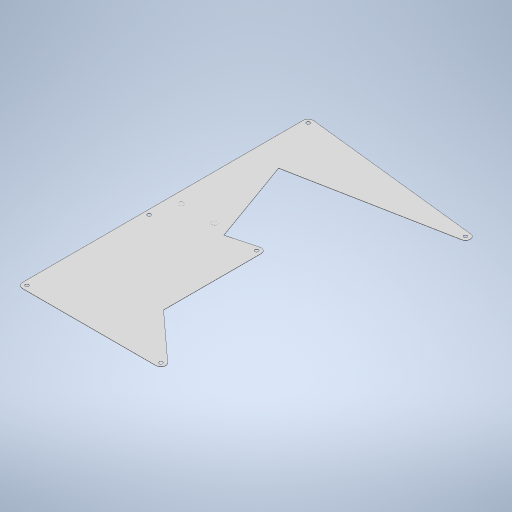
# Autodesk Inventor part: base_main_pcb_full
Saved by Autodesk Inventor 2024 (Build 280153000, 153)
## iProperties
Created: 2026-03-21
Part Number: base_main_pcb_full
Material: Generic
Document SubType Name: Modeling
Designer: schar
Density: 1 g/cm^3
Appearance: Default
Author: schar
Autodesk Inventor part; units mm, degrees
ref_plane "YZ Plane" through (0, 0, 0) normal (1, 0, 0) x (0, 1, 0)
ref_plane "Work Plane1" through (-205, 0.2, 0) normal (0, 1, 0) x (1, 0, 0)
sketch "Sketch1" plane through (-205, 0.2, 0) normal (0, 1, 0) x (1, 0, 0)
  circle A0 centre (172.5, -37.3) radius 1.675 projected
  circle A1 centre (172.5, -37.3) radius 4.5
  circle A2 centre (172.5, -37.3) radius 1.675
  circle A3 centre (7.5, -19) radius 1.675 projected
  circle A4 centre (7.5, -19) radius 4.5
  circle A5 centre (7.5, -19) radius 1.675
  circle A6 centre (86.5, -146.2) radius 1.675 projected
  circle A7 centre (86.5, -146.2) radius 4.5
  circle A8 centre (86.5, -146.2) radius 1.675
  circle A9 centre (7.5, -167.45) radius 1.675 projected
  circle A10 centre (7.5, -167.45) radius 4.5
  circle A11 centre (7.5, -167.45) radius 1.675
  circle A12 centre (7.5, -281.46) radius 1.675 projected
  circle A13 centre (7.5, -281.46) radius 4.5
  circle A14 centre (7.5, -281.46) radius 1.675
  circle A15 centre (132.5, -281.46) radius 1.675 projected
  circle A16 centre (132.5, -281.46) radius 4.5
  circle A17 centre (132.5, -281.46) radius 1.675
  line L0 (132.5, -285.96) -> (7.5, -285.96)
  line L1 (3, -281.46) -> (3, -167.45)
  line L2 (135.7704, -278.369) -> (10.5327, -164.1254)
  line L3 (91, -146.2) -> (91, -237.5288)
  line L4 (84.825, -142.0234) -> (6.3328, -163.104)
  line L5 (91, -237.5288) -> (10.5327, -164.1254)
  line L6 (12, -19) -> (58.7973, -149.0136)
  line L7 (3, -19) -> (3, -167.45)
  line L8 (172.5, -41.8) -> (30.084, -69.2416)
  line L9 (172.5, -32.8) -> (8.061, -14.5351)
  point P0 (205, 0)
  dimension "d1" = 9
  dimension "d2" = 9
  dimension "d3" = 9
  dimension "d4" = 9
  dimension "d5" = 9
  dimension "d6" = 9
  constraints: 20 end point, 14 point on circle, 12 centre point, 12 coincident, 6 tangent, 2 point on line, 1 concentric, 1 parallel, 1 perpendicular, 1 vertical
  measures "d1" diameter of A1
  measures "d2" diameter of A4
  measures "d3" diameter of A7
  measures "d4" diameter of A10
  measures "d5" diameter of A13
  measures "d6" diameter of A16
extrude "Extrusion1" add sketch "Sketch1" along normal blind 0.2 contours A1 | A1 L8 L6 A4 L9 | A4 | L6 L4 A10 L7 A4 | L4 A7 L3 L2 A10 | A10 | A10 L2 A16 L0 A13 L1 | A7 | A13 | A16 L2 picked at (134.365, -278.4554)
ref_plane "Work Plane2" through (-205, 0.4, 0) normal (0, 1, 0) x (1, 0, 0)
sketch "Sketch3" plane through (-205, 0.2, 0) normal (0, -1, 0) x (1, 0, 0)
  line L0 (3, 19) -> (3, 281.46) projected
  line L1 (3, 143.5142) -> (56.8178, 143.5142)
  line L2 (58.7973, 149.0136) -> (30.084, 69.2416) projected
  circle A0 centre (13.4848, 143.5142) radius 2.5
  circle A1 centre (44.4406, 143.5142) radius 2.5
  point P0 (205, 0)
  dimension "d11" = 5
  dimension "d12" = 5
  constraints: 4 point on line, 2 centre point, 2 end point, 1 horizontal
  measures "d11" diameter of A0
  measures "d12" diameter of A1
extrude "Extrusion2" add sketch "Sketch3" along normal blind 1
body "Solid2"
